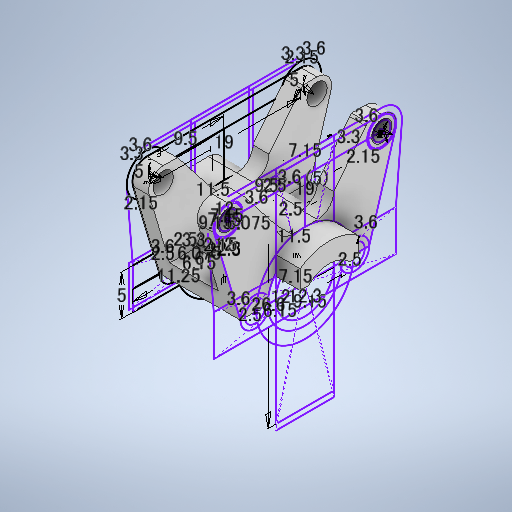
# Autodesk Inventor part: ikafly6.0_2.5cl
Saved by Autodesk Inventor 2025 (Build 290162000, 162)
## iProperties
Created: 2024-06-20
Part Number: ikafly6.0_2.5cl
Material: 一般
Document SubType Name: Modeling
Designer: Saigusa
Density: 1 g/cm^3
Appearance: 既定
Author: Saigusa
Autodesk Inventor part; units mm, degrees
ref_plane "YZ Plane" through (0, 0, 0) normal (1, 0, 0) x (0, 1, 0)
ref_plane "XZ Plane" through (0, 0, 0) normal (0, 1, 0) x (-1, 0, 0)
ref_plane "XY Plane" through (0, 0, 0) normal (0, 0, 1) x (1, 0, 0)
sketch "スケッチ1" plane through (0, 0, 0) normal (1, 0, 0) x (0, 1, 0)
  circle A0 centre (0, 0) radius 4.575
  circle A1 centre (0, 0) radius 3.575
  line L0 (0, 0) -> (0, 6)
  line L1 (0, 6) -> (0, -6)
  line L2 (0, 0) -> (11.5, 0)
  line L3 (11.5, 0) -> (11.5, 9.5)
  line L4 (11.5, 9.5) -> (11.5, -9.5)
  circle A2 centre (11.5, 9.5) radius 1.65
  circle A3 centre (11.5, -9.5) radius 1.65
  line L5 (0, 0) -> (0, 11.25)
  line L6 (0, 11.25) -> (0, -11.25)
  line L7 (-2.5, -11.25) -> (2.5, -11.25)
  line L8 (2.5, -11.25) -> (2.5, 11.25)
  line L9 (2.5, 11.25) -> (-2.5, 11.25)
  line L10 (-2.5, 11.25) -> (-2.5, -11.25)
  line L11 (-2.5, -11.25) -> (2.5, 11.25) construction
  line L12 (2.5, -11.25) -> (-2.5, 11.25) construction
  circle A4 centre (11.5, 9.5) radius 2.5
  circle A5 centre (11.5, -9.5) radius 2.5
  line L13 (2.5, 11.25) -> (11.2899, 11.9912)
  line L14 (2.5, -11.25) -> (11.2899, -11.9912)
  line L15 (14, 9.5) -> (14, -9.5)
  line L16 (0, -3.575) -> (14, -3.575)
  line L17 (0, 3.575) -> (14, 3.575)
  circle A6 centre (0, 0) radius 6
  line L18 (0, 0) -> (0, 6.15)
  line L19 (0, 6.15) -> (0, -6.15)
  circle A7 centre (0, 6.15) radius 1.25
  circle A8 centre (0, -6.15) radius 1.25
  line L20 (0, 0) -> (0, -6.075)
  line L21 (0, 0) -> (0, 6.075)
  circle A9 centre (0, -6.075) radius 1.25
  circle A10 centre (0, 6.075) radius 1.25
  circle A11 centre (11.5, 9.5) radius 1.075
  circle A12 centre (11.5, -9.5) radius 1.075
  circle A13 centre (11.5, -9.5) radius 1.8
  circle A14 centre (11.5, 9.5) radius 1.8
  line L22 (11.5, -9.5) -> (13.3, -9.5)
  line L23 (11.5, 9.5) -> (13.3, 9.5)
  line L24 (13.3, -9.5) -> (13.3, 9.5)
  circle A15 centre (0, -6.15) radius 1.8
  circle A16 centre (0, 6.15) radius 1.8
  line L25 (0, -7.95) -> (10.9858, -11.225)
  line L26 (0, 7.95) -> (10.9858, 11.225)
  point P0 (0, 4.575)
  point P1 (0, -4.575)
  point P2 (2.5, 3.575)
  point P3 (2.5, 2.5555)
  point P4 (2.5, -2.5555)
  point P5 (2.5, -3.575)
  point P6 (0, 7.4)
  point P7 (0, 4.9)
  point P8 (0, -4.9)
  point P9 (0, -7.4)
  point P10 (2.5, 5.4544)
  point P11 (2.5, -5.4544)
  point P12 (4.8186, 3.575)
  point P13 (4.8186, -3.575)
  point P14 (2.8548, 3.575)
  point P15 (2.8548, -3.575)
  point P16 (0, 7.95)
  point P17 (2.5, -8.6953)
  point P18 (2.5, 8.6953)
  dimension "d114" = 3.6
  dimension "d115" = 3.6
  dimension "d0" = 9.15
  dimension "d1" = 7.15
  dimension "d2" = 6
  dimension "d3" = 12
  dimension "d6" = 11.5
  dimension "d7" = 9.5
  dimension "d8" = 19
  dimension "d9" = 3.3
  dimension "d10" = 3.3
  dimension "d11" = 11.25
  dimension "d12" = 22.5
  dimension "d13" = 5
  dimension "d14" = 5
  dimension "d15" = 5
  dimension "d28" = 12
  dimension "d29" = 6.15
  dimension "d30" = 12.3
  dimension "d31" = 2.5
  dimension "d32" = 2.5
  dimension "d99" = 6.075
  dimension "d100" = 6.075
  dimension "d101" = 2.5
  dimension "d102" = 2.5
  dimension "d110" = 2.15
  dimension "d111" = 2.15
  dimension "d112" = 3.6
  dimension "d113" = 3.6
  constraints: 54 end point, 17 coincident, 15 centre point, 12 point on line, 10 point on circle, 7 tangent, 4 perpendicular, 3 horizontal, 3 parallel, 2 midpoint, 2 vertical alignment, 1 vertical, 4 other
  measures "d0" diameter of A0
  measures "d1" diameter of A1
  measures "d2" distance of L0.start L0.end
  measures "d3" distance of L0.end L1.end
  measures "d6" distance of L0.start L2.end
  measures "d7" distance of L2.end L3.end
  measures "d8" distance of L3.end L4.end
  measures "d9" diameter of A2
  measures "d10" diameter of A3
  measures "d11" distance of L0.start L5.end
  measures "d12" distance of L5.end L6.end
  measures "d13" distance of L9.end L8.end
  measures "d14" diameter of A4
  measures "d15" diameter of A5
  measures "d28" diameter of A6
  measures "d29" distance of L18.start L18.end
  measures "d30" distance of L18.end L19.end
  measures "d31" diameter of A7
  measures "d32" diameter of A8
  measures "d99" distance of L18.start L20.end
  measures "d100" distance of L18.start L21.end
  measures "d101" diameter of A9
  measures "d102" diameter of A10
  measures "d110" diameter of A11
  measures "d111" diameter of A12
  measures "d112" diameter of A13
  measures "d113" diameter of A14
extrude "押し出し7" add sketch "スケッチ1" along normal blind 2 contours L2 A6 L16 A0 | A0 L17 A6 L2 | A0 L8 A6 L17 | L16 A6 L8 A0 | A6 L17 L3 L2 | L2 L4 L16 A6 | A0 A16 A6 L8 | A6 L8 L26 A4 L3 L17 | L8 A6 A15 A0 | L16 L4 A5 L25 L8 A6 | L3 L17 L24 L16 L4 | A0 L0 A10 A6 A16 | A6 A16 L26 L8 | L3 A4 L24 L17 | A15 A6 A9 L1 A0 | L8 L25 A15 A6 | L16 L24 A5 L4 | A6 A10 L5 A16 | A4 L26 A14 L3 | L3 A14 L24 A4 | A15 L6 A8 A6 | A5 L24 A13 L4 | L4 A13 L25 A5 | L0 A7 A6 A10 | A14 L23 A2 L3 | L3 A2 L23 A14 | A9 A6 A8 L1 | A13 L22 A3 L4 | L4 A3 L22 A13 picked at (1.3383, 5.2331) picked at (1.3383, -5.2331) picked at (0.0969, 4.8614) picked at (0.0969, -4.8614)
extrude "押し出し8" add sketch "スケッチ1" along normal blind 10 contours L2 A6 L16 A0 | A0 L17 A6 L2 | A0 L8 A6 L17 | L16 A6 L8 A0 | A6 L17 L3 L2 | L2 L4 L16 A6 | A0 A16 A6 L8 | L8 A6 A15 A0 | L3 L17 L24 L16 L4 | A0 L0 A10 A6 A16 | A6 A16 L26 L8 | A15 A6 A9 L1 A0 | L8 L25 A15 A6 | A6 A10 L5 A16 | L17 L15 L16 L24 | A15 L6 A8 A6 | L0 A7 A6 A10 | A6 L5 A10 | A9 A6 A8 L1 | L0 A6 A7 | A8 A6 L1 | A8 L6 A6 picked at (1.3383, 5.2331) picked at (1.3383, -5.2331) picked at (0.0969, 4.8614) picked at (0.0969, -4.8614) picked at (0.2292, 5.6392) picked at (0.2292, -5.6392)
sketch "スケッチ6" plane through (10, 0, 0) normal (1, 0, 0) x (0, 0, -1)
  line L0 (0, 0) -> (-6.15, 0)
  line L1 (-6.15, 0) -> (6.15, 0)
  circle A0 centre (-6.15, 0) radius 1.25
  circle A1 centre (6.15, 0) radius 1.25
  line L2 (-11.25, 2.5) -> (11.25, 2.5)
  line L3 (11.25, 2.5) -> (11.25, -2.5)
  line L4 (11.25, -2.5) -> (-11.25, -2.5)
  line L5 (-11.25, -2.5) -> (-11.25, 2.5)
  line L6 (-11.25, 2.5) -> (11.25, -2.5) construction
  line L7 (11.25, 2.5) -> (-11.25, -2.5) construction
  line L8 (0, 0) -> (0, 11.5)
  line L9 (0, 11.5) -> (-9.5, 11.5)
  line L10 (-9.5, 11.5) -> (9.5, 11.5)
  circle A2 centre (-9.5, 11.5) radius 1.65
  circle A3 centre (9.5, 11.5) radius 1.65
  circle A4 centre (0, 0) radius 6
  circle A5 centre (0, 0) radius 4.575
  arc A6 (11.9912, 11.2899) -> (9.5, 14) centre (9.5, 11.5) ccw
  line L11 (11.25, 2.5) -> (11.9912, 11.2899)
  line L12 (-11.25, 2.5) -> (-11.9912, 11.2899)
  line L13 (-9.5, 14) -> (9.5, 14)
  circle A7 centre (0, 0) radius 3.575
  line L14 (-3.575, 14) -> (-3.575, 4.8186)
  line L15 (3.575, -14) -> (-3.575, -14)
  line L16 (-3.575, 14) -> (3.575, 14)
  line L17 (3.575, 14) -> (3.575, -14)
  line L18 (3.575, -14) -> (-3.575, 14) construction
  line L19 (-3.575, -14) -> (3.575, 14) construction
  circle A8 centre (-9.5, 11.5) radius 1.075
  circle A9 centre (9.5, 11.5) radius 1.075
  circle A10 centre (9.5, 11.5) radius 1.8
  circle A11 centre (-9.5, 11.5) radius 1.8
  line L20 (-9.5, 11.5) -> (-9.5, 13.3)
  line L21 (-9.5, 13.3) -> (9.5, 13.3)
  circle A12 centre (-6.15, 0) radius 1.8
  circle A13 centre (6.15, 0) radius 1.8
  line L22 (-7.95, 0) -> (-11.225, 10.9858)
  line L23 (4.575, 0) -> (7.95, 0)
  line L24 (7.95, 0) -> (11.225, 10.9858)
  line L25 (3.575, -13.3) -> (-3.575, -13.3)
  line L26 (-3.575, -13.3) -> (-3.575, 13.3)
  line L27 (-3.575, 13.3) -> (3.575, 13.3)
  line L28 (3.575, 13.3) -> (3.575, -13.3)
  line L29 (3.575, -13.3) -> (-3.575, 13.3) construction
  line L30 (-3.575, -13.3) -> (3.575, 13.3) construction
  point P0 (-5.4544, 2.5)
  point P1 (5.4544, 2.5)
  point P2 (-3.575, 11.5)
  point P3 (-2.5555, 2.5)
  point P4 (2.5555, 2.5)
  point P5 (3.575, 2.5)
  point P6 (3.575, 11.5)
  point P7 (-8.6953, 2.5)
  point P8 (8.6953, 2.5)
  point P9 (3.575, 0)
  point P10 (-3.575, 11.5)
  point P11 (3.575, -2.5)
  point P12 (0, 2.5)
  point P13 (0, 3.575)
  point P14 (3.575, 4.8186)
  point P15 (-3.575, 4.8186)
  point P16 (-3.575, 2.5)
  dimension "d69" = 12
  dimension "d120" = 3.6
  dimension "d121" = 3.6
  dimension "d56" = 6.15
  dimension "d57" = 12.3
  dimension "d58" = 2.5
  dimension "d59" = 2.5
  dimension "d62" = 11.5
  dimension "d63" = 9.5
  dimension "d64" = 19
  dimension "d65" = 3.3
  dimension "d67" = 3.3
  dimension "d70" = 9.15
  dimension "d79" = 7.15
  dimension "d116" = 2.15
  dimension "d117" = 2.15
  dimension "d118" = 3.6
  dimension "d119" = 3.6
  dimension "d124" = 7.15
  dimension "d125" = 26.6
  constraints: 62 end point, 13 coincident, 11 centre point, 6 midpoint, 6 point on circle, 5 horizontal, 5 parallel, 4 tangent, 3 perpendicular, 2 horizontal alignment, 2 point on line, 2 vertical, 5 other
  measures "d56" distance of L0.start L0.end
  measures "d57" distance of L0.end L1.end
  measures "d58" diameter of A0
  measures "d59" diameter of A1
  measures "d62" distance of L0.start L8.end
  measures "d63" distance of L8.end L9.end
  measures "d64" distance of L9.end L10.end
  measures "d65" diameter of A2
  measures "d67" diameter of A3
  measures "d70" diameter of A5
  measures "d79" diameter of A7
  measures "d116" diameter of A8
  measures "d117" diameter of A9
  measures "d118" diameter of A10
  measures "d119" diameter of A11
  measures "d124" distance of L26.end L27.end
  measures "d125" distance of L25.end L26.end
extrude "押し出し9" add sketch "スケッチ6" against normal blind 2 contours L2 L22 A11 L9 L14 A4 | L14 L9 L8 A4 | A4 L17 L10 A10 L24 L2 | A4 L8 L10 L17 | L14 L21 L17 L10 L9 | L9 A11 L21 L14 | L17 L21 A10 L10 | A11 L20 A2 L9 | L9 A2 L20 A11 | A10 | A2 L20 A8 L9 | L9 A8 L20 A2 | A3
extrude "押し出し10" add sketch "スケッチ1" against normal blind 0.5 contours L2 A6 L16 A0 | A0 L17 A6 L2 | A6 L17 L3 L2 | L2 L4 L16 A6 | L3 L17 L24 L16 L4 | L17 L15 L16 L24
sketch "スケッチ7" plane through (-0.5, 0, 0) normal (-1, 0, 0) x (0, 0, 1)
  circle A0 centre (0, 0) radius 3.575
  line L0 (-9.5, 14) -> (9.5, 14)
  line L1 (-3.575, 14) -> (3.575, 14)
  circle A1 centre (0, 0) radius 4.575
  line L2 (-11.25, 0) -> (-11.25, 2.5)
  line L3 (11.25, -2.5) -> (-11.25, -2.5)
  line L4 (-11.25, -2.5) -> (-11.25, 2.5)
  line L5 (-11.25, 2.5) -> (11.25, 2.5)
  line L6 (11.25, 2.5) -> (11.25, -2.5)
  line L7 (11.25, -2.5) -> (-11.25, 2.5) construction
  line L8 (-11.25, -2.5) -> (11.25, 2.5) construction
  line L9 (-3.575, 14) -> (-3.575, 0)
  line L10 (3.575, 14) -> (3.575, 0)
  point P0 (-3.575, 2.5)
  point P1 (-2.5555, 2.5)
  point P2 (2.5555, 2.5)
  point P3 (3.575, 2.5)
  dimension "d75" = 7.15
  dimension "d76" = 5
  constraints: 22 end point, 2 centre point, 2 coincident, 2 midpoint, 2 parallel, 2 point on circle, 2 point on line, 2 tangent, 1 horizontal, 1 perpendicular
  measures "d75" diameter of A0
  measures "d76" distance of L3.end L2.end
extrude "押し出し11" add sketch "スケッチ7" along normal blind 3 contours A0 L5 L9 A1 L10 | A1 L9 L0 L10
extrude "押し出し12" add sketch "スケッチ6" along normal blind 3 contours L2 L26 A5 L8 A7 | A7 L8 A5 L17 L2 | L26 A4 L8 A5 | A5 L8 A4 L17
sketch "スケッチ8" plane through (13, 0, 0) normal (1, 0, 0) x (0, 0, -1)
  line L0 (-3.575, 2.5) -> (-3.575, 14) projected
  line L1 (3.575, 14) -> (3.575, 2.5) projected
  line L2 (-3.575, 14) -> (3.575, 14)
  line L3 (3.575, 14) -> (3.575, 2.5)
  line L4 (3.575, 2.5) -> (-3.575, 2.5)
  line L5 (-3.575, 2.5) -> (-3.575, 14)
  circle A0 centre (0, 0) radius 6
  line L6 (-3.575, 14) -> (3.575, 14)
  line L7 (3.575, 14) -> (3.575, 6)
  line L8 (3.575, 6) -> (-3.575, 6)
  line L9 (-3.575, 6) -> (-3.575, 14)
  dimension "d89" = 12
  constraints: 16 end point, 4 parallel, 2 horizontal, 2 perpendicular, 1 centre point, 1 coincident, 1 point on line
  measures "d89" diameter of A0
extrude "押し出し13" cut sketch "スケッチ8" against normal blind 16.5 contours L0 L2 L1 L8
fillet "フィレット1" radius 2 8 edges at (9, 6, 3.575) (9, 6, -3.575) (1, 6, -3.575) (5, 6, 3.575) (5, 6, -3.575) (1, 6, 3.575) (-1.75, 6, 3.575) (-1.75, 6, -3.575)
sketch "スケッチ9" plane through (10, 0, 0) normal (1, 0, 0) x (0, 0, -1)
  arc A0 (2.5555, 2.5) -> (-2.5555, 2.5) centre (0, 0) ccw projected
  line L0 (0, 0) -> (0, 11.5)
  line L1 (0, 11.5) -> (-9.5, 11.5)
  circle A1 centre (9.5, 11.5) radius 1.65 projected
  line L2 (-9.5, 11.5) -> (9.5, 11.5)
  circle A2 centre (-9.5, 11.5) radius 2.5
  circle A3 centre (9.5, 11.5) radius 2.5
  arc A4 (-3.575, 8) -> (-1.575, 6) centre (-1.575, 8) ccw
  line L3 (-3.575, 8) -> (-7.5334, 13.0435)
  arc A5 (1.575, 6) -> (3.575, 8) centre (1.575, 8) ccw
  line L4 (3.575, 8) -> (7.5334, 13.0435)
  line L5 (9.5, 14) -> (3.575, 14)
  line L6 (-3.575, 8) -> (3.575, 8)
  line L7 (3.575, 8) -> (3.575, 14)
  line L8 (3.575, 14) -> (-3.575, 14)
  line L9 (-3.575, 14) -> (-3.575, 8)
  line L10 (-3.575, 8) -> (-9.5, 8)
  line L11 (-9.5, 8) -> (-9.5, 14)
  line L12 (-9.5, 14) -> (-3.575, 14)
  line L13 (-3.575, 14) -> (-3.575, 8)
  line L14 (3.575, 8) -> (9.5, 8)
  line L15 (9.5, 8) -> (9.5, 14)
  line L16 (9.5, 14) -> (3.575, 14)
  line L17 (3.575, 14) -> (3.575, 8)
  dimension "d93" = 11.5
  dimension "d94" = 9.5
  dimension "d95" = 5
  dimension "d96" = 5
  constraints: 36 end point, 7 point on circle, 6 parallel, 4 centre point, 4 perpendicular, 3 horizontal, 2 coincident, 2 tangent, 1 vertical
  measures "d93" distance of L0.start L0.end
  measures "d94" distance of L0.end L1.end
  measures "d95" diameter of A2
  measures "d96" diameter of A3
extrude "押し出し14" cut sketch "スケッチ9" against normal blind 16.5 contours L3 L1 L9 | L7 L2 L4 | L1 L3 A2 L12 L9 | L7 L5 A3 L4 L2
hole "穴2" at (0, 0, 6.075) at (0, 0, -6.075) direction (1, 0, 0) diameter 2.45 depth 2
extrude "押し出し15" add sketch "スケッチ1" along normal blind 2 contours A2 L23 A11 L3 | L3 A11 L23 A2 | A3 L22 A12 L4 | L4 A12 L22 A3
hole "穴3" at (10, 11.5, 9.5) at (10, 11.5, -9.5) direction (-1, 0, 0) diameter 2.5 end through all
